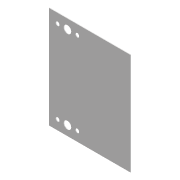
# Autodesk Inventor part: Part78
Saved by Autodesk Inventor 2020.5 (Build 245400000, 400)
## iProperties
Created: 2022-11-26
Part Number: Part78
Material: 一般
Document SubType Name: Modeling
Designer: Administrator
Density: 1 g/cm^3
Appearance: 既定
Author: Administrator
Autodesk Inventor part; units mm, degrees
ref_plane "YZ Plane" through (0, 0, 0) normal (1, 0, 0) x (0, 1, 0)
ref_plane "XZ Plane" through (0, 0, 0) normal (0, 1, 0) x (-1, 0, 0)
ref_plane "XY Plane" through (0, 0, 0) normal (0, 0, 1) x (1, 0, 0)
sketch "スケッチ1" plane through (0, 0, 0) normal (0, 0, 1) x (1, 0, 0)
  circle A0 centre (-15.5, 0) radius 2.5 projected
  circle A1 centre (15.5, 0) radius 2.5 projected
  circle A2 centre (0, 0) radius 11 projected
  line L0 (-15.1987, 13) -> (15.1987, 13) projected
  arc A3 (15.1987, -13) -> (15.1987, 13) centre (0, 0) ccw projected
  line L1 (15.1987, -13) -> (-15.1987, -13) projected
  arc A4 (-15.1987, 13) -> (-15.1987, -13) centre (0, 0) ccw projected
  circle A5 centre (-15.5, -130.182) radius 2.5 projected
  circle A6 centre (15.5, -130.182) radius 2.5 projected
  circle A7 centre (0, -130.182) radius 11 projected
  line L2 (-15.1987, -143.182) -> (15.1987, -143.182) projected
  arc A8 (-15.1987, -117.182) -> (-15.1987, -143.182) centre (0, -130.182) ccw projected
  line L3 (15.1987, -117.182) -> (-15.1987, -117.182) projected
  arc A9 (15.1987, -143.182) -> (15.1987, -117.182) centre (0, -130.182) ccw projected
  circle A10 centre (0, -130.182) radius 5 projected
  circle A11 centre (0, 0) radius 5 projected
  line L4 (-29, -63.3408) -> (-16.25, -63.3408) projected
  arc A12 (-16.25, -63.3408) -> (-16.25, -33.3408) centre (-16.25, -48.3408) ccw projected
  line L5 (-16.25, -33.3408) -> (-29, -33.3408) projected
  line L6 (-29, -33.3408) -> (-29, 14.909) projected
  line L7 (119, 14.909) -> (-29, 14.909) projected
  line L8 (119, 14.909) -> (119, -145.0901) projected
  line L9 (119, -145.0901) -> (-29, -145.0901) projected
  circle A13 centre (14.75, -81.8408) radius 15 projected
  circle A14 centre (15.5, 0.0009) radius 3 projected
  circle A15 centre (15.5, -130.1819) radius 3 projected
  circle A16 centre (-15.5, 0.0009) radius 3 projected
  circle A17 centre (0, -130.1819) radius 6 projected
  circle A18 centre (-15.5, -130.1819) radius 3 projected
  circle A19 centre (0, 0.0009) radius 6 projected
  line L10 (-29, -63.3408) -> (-29, -33.3408)
  line L11 (119, 16.9081) -> (119, 16.909) projected
  line L12 (119, -145.0901) -> (119, 14.909)
  line L13 (119, 14.909) -> (119, 14.909)
  line L14 (119, 14.909) -> (119, -145.0901)
  line L15 (119, -145.0901) -> (119, -145.0901)
  circle A20 centre (0, -130.1819) radius 55
  circle A21 centre (0, 0.0009) radius 55
  line L16 (119, -145.0901) -> (59, -145.0901)
  line L17 (59, -145.0901) -> (59, 14.909)
  line L18 (59, 14.909) -> (119, 14.909)
  line L19 (119, 14.909) -> (119, -145.0901)
  line L20 (-29, -145.0901) -> (-29, -63.3408) projected
  point P0 (0, 0)
  dimension "d2" = 110
  dimension "d3" = 110
  dimension "d4" = 60
  dimension "d5" = 159.9991
  constraints: 18 end point, 5 equal length, 2 centre point, 2 coincident, 2 perpendicular, 1 point on line, 1 vertical
  measures "d2" diameter of A20
  measures "d3" diameter of A21
  measures "d4" distance of L14.end L16.end
  measures "d5" distance between parallel lines of L18 L16
extrude "押し出し1" add sketch "スケッチ1" along normal blind 1 contours A2 | L0 A3 L1 A4 | A7 | A8 L3 A9 L2 | L10 A21 A12 L4 | L4 A12 A21 L7 L17 L9 A20 A13 L20 | L10 L5 A12 A21 | A20 A13 L9 L20 | A12 L5 L6 L7 A21 | A20 A13 | A13 A20 | L7 L8 L9 L17
